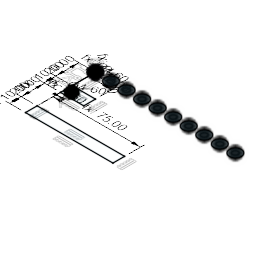
Initial_Gears (Autodesk Fusion 360 design; units mm, degrees)
part number: 2026-02-16-14-12-18-314
Autodesk Fusion 360 part; units mm, degrees
(part 1 of 40)
sketch "Crank Slider 2" plane through (0, 0, 0) normal (0, 1, 0) x (1, 0, 0)
  circle A0 centre (0, 0) radius 60
  circle A1 centre (0, 0) radius 50 construction
  line L0 (0, 0) -> (0, 50) construction
  circle A2 centre (0, 50) radius 2.3
  circle A3 centre (0, 0) radius 2.3
  line L1 (0, 0) -> (100, 0) construction
  line L2 (130, 5) -> (70, 5)
  line L3 (70, 5) -> (70, -5)
  line L4 (70, -5) -> (130, -5)
  line L5 (130, -5) -> (130, 5)
  line L6 (130, 5) -> (70, -5) construction
  line L7 (70, 5) -> (130, -5) construction
  line L8 (100, 0) -> (75, 0) construction
  line L9 (100, 0) -> (125, 0) construction
  circle A4 centre (75, 0) radius 2.3
  circle A5 centre (125, 0) radius 2.3
  line L10 (100, 0) -> (250, 0) construction
  line L11 (330, 5) -> (170, 5)
  line L12 (170, 5) -> (170, -5)
  line L13 (170, -5) -> (330, -5)
  line L14 (330, -5) -> (330, 5)
  line L15 (330, 5) -> (170, -5) construction
  line L16 (170, 5) -> (330, -5) construction
  line L17 (250, 0) -> (175, 0) construction
  line L18 (250, 0) -> (325, 0) construction
  circle A6 centre (175, 0) radius 2.3
  circle A7 centre (325, 0) radius 2.3
  line L19 (325, 0) -> (375, 0) construction
  line L20 (365, 5) -> (385, 5)
  line L21 (385, 5) -> (385, -5)
  line L22 (385, -5) -> (365, -5)
  line L23 (365, -5) -> (365, 5)
  line L24 (365, 5) -> (385, -5) construction
  line L25 (385, 5) -> (365, -5) construction
  line L26 (375, 0) -> (525, 0) construction
  line L27 (637.5, 5) -> (412.5, 5)
  line L28 (412.5, 5) -> (412.5, -5)
  line L29 (412.5, -5) -> (637.5, -5)
  line L30 (637.5, -5) -> (637.5, 5)
  line L31 (637.5, 5) -> (412.5, -5) construction
  line L32 (412.5, 5) -> (637.5, -5) construction
  line L33 (412.5, 5) -> (637.5, 5)
  line L34 (637.5, 5) -> (637.5, 15)
  line L35 (637.5, 15) -> (412.5, 15)
  line L36 (412.5, 15) -> (412.5, 5)
  line L37 (412.5, -15) -> (412.5, -5)
  line L38 (637.5, -15) -> (412.5, -15)
  line L39 (637.5, -5) -> (637.5, -15)
  circle A8 centre (375, 0) radius 2.3
  line L40 (271.0638, 125.2182) -> (271.2213, 125.2035) construction
  line L41 (271.2213, 125.2035) -> (271.3791, 125.1902) construction
  point P0 (100, 0)
  point P1 (250, 0)
  point P2 (375, 0)
  point P3 (525, 0)
  dimension "d1" = 120
  dimension "d4" = 100
  dimension "d6" = 4.6
  dimension "d7" = 4.6
  dimension "d8" = 100
  dimension "d11" = 60
  dimension "d12" = 10
  dimension "d13" = 25
  dimension "d14" = 25
  dimension "d15" = 4.6
  dimension "d16" = 4.6
  dimension "d18" = 150
  dimension "d20" = 160
  dimension "d21" = 10
  dimension "d22" = 75
  dimension "d23" = 75
  dimension "d24" = 4.6
  dimension "d25" = 4.6
  dimension "d26" = 50
  dimension "d27" = 20
  dimension "d28" = 10
  dimension "d29" = 150
  dimension "d30" = 225
  dimension "d31" = 10
  dimension "d32" = 225
  dimension "d33" = 10
  dimension "d34" = 4.6
  constraint coincident A0.centre A1.centre
  constraint coincident A1 L0.end
  constraint vertical L0
  constraint coincident L0.end A2.centre
  constraint concentric A0 A3
  constraint perpendicular L0 L1
  constraint horizontal L2
  constraint perpendicular L2 L3
  constraint parallel L2 L4
  constraint parallel L3 L5
  constraint coincident L6 P0
  constraint coincident L7 P0
  constraint coincident P0 L1.end
  constraint parallel L1 L8
  constraint parallel L8 L9
  constraint coincident L8.end A4.centre
  constraint coincident L9.end A5.centre
  constraint parallel L9 L10
  constraint horizontal L11
  constraint perpendicular L11 L12
  constraint parallel L11 L13
  constraint parallel L12 L14
  constraint coincident L15 P1
  constraint coincident L16 P1
  constraint coincident P1 L10.end
  constraint parallel L10 L17
  constraint parallel L10 L18
  constraint coincident L17.end A6.centre
  constraint coincident L18.end A7.centre
  constraint parallel L18 L19
  constraint horizontal L20
  constraint perpendicular L20 L21
  constraint parallel L20 L22
  constraint parallel L21 L23
  constraint coincident L24 P2
  constraint coincident L25 P2
  constraint coincident P2 L19.end
  constraint perpendicular L21 L26
  constraint horizontal L27
  constraint perpendicular L27 L28
  constraint parallel L27 L29
  constraint parallel L28 L30
  constraint coincident L31 P3
  constraint coincident L32 P3
  constraint coincident P3 L26.end
  constraint horizontal L33
  constraint vertical L34
  constraint horizontal L35
  constraint vertical L36
  constraint symmetric L26 L27.end L28.end
  constraint symmetric L26 L27.start L29.end
  constraint symmetric L26 L34.end L38.start
  constraint symmetric L26 L35.end L37.start
  measures "d1" diameter of A0
  measures "d4" diameter of A1
  measures "d6" diameter of A2
  measures "d7" diameter of A3
  measures "d8" distance of A0.centre P0
  measures "d11" distance of L3.end L4.end
  measures "d12" distance of L2.end L3.end
  measures "d13" distance of P0 L8.end
  measures "d14" distance of P0 L9.end
  measures "d15" diameter of A4
  measures "d16" diameter of A5
  measures "d18" distance of P0 P1
  measures "d20" distance of L12.end L13.end
  measures "d21" distance of L11.end L12.end
  measures "d22" distance of P1 L17.end
  measures "d23" distance of P1 L18.end
  measures "d24" diameter of A6
  measures "d25" diameter of A7
  measures "d26" distance of L18.end P2
  measures "d27" distance of L21.end L22.end
  measures "d28" distance of L20.end L21.end
  measures "d29" distance of P2 P3
  measures "d30" distance of L28.end L29.end
  measures "d31" distance of L27.end L28.end
  measures "d32" distance of L27.end L27.start
  measures "d33" distance of L27.end L35.end
  measures "d34" diameter of A8
extrude "Extrude1" add sketch "Crank Slider 2" along normal blind 4.2 makes body 1 at (274.7199, 0, 4.047) makes body 2 at (108.0532, 0, -4.047) makes body 3 at (367.5667, 0, 0) makes body 4 at (-13.4258, 0, -32.3033) makes body 5 at (487.5, 0, 5)
sketch "Sketch2" plane through (0, 0, 0) normal (0, 1, 0) x (1, 0, 0)
  line L0 (0, 0) -> (212.132, 0) construction
  line L1 (212.132, 0) -> (212.132, 150) construction
  line L2 (212.132, 150) -> (0, 0) construction
  line L3 (0, 0) -> (-50, 0) construction
  line L4 (-50, 0) -> (-50, -100) construction
  line L5 (-50, -100) -> (250, -100)
  line L6 (250, -100) -> (250, 200)
  line L7 (250, 200) -> (-50, 200)
  line L8 (-50, 200) -> (-50, -100)
  circle A0 centre (212.132, 150) radius 2.3
  circle A1 centre (212.132, 0) radius 2.3
  circle A2 centre (0, 0) radius 2.3
  line L9 (0, 0) -> (106.066, 75) construction
  circle A3 centre (106.066, 75) radius 2.3
  dimension "d41" = 212.132
  dimension "d42" = 150
  dimension "d43" = 259.8076
  dimension "d44" = 50
  dimension "d45" = 100
  dimension "d46" = 300
  dimension "d47" = 300
  dimension "d48" = 4.6
  dimension "d49" = 4.6
  dimension "d50" = 4.6
  dimension "d74" = 4.6
  constraint coincident L0.start L2.end
  constraint horizontal L0
  constraint perpendicular L0 L1
  constraint parallel L0 L3
  constraint perpendicular L3 L4
  constraint horizontal L5
  constraint vertical L6
  constraint horizontal L7
  constraint vertical L8
  constraint coincident L1.end L2.start
  constraint coincident L0.end L1.start
  constraint midpoint L2 L9.end
  constraint coincident L9.end A3.centre
  measures "d41" distance of L0.start L0.end
  measures "d42" distance of L0.end L1.end
  measures "d43" distance of L1.end L0.start
  measures "d44" distance of L0.start L3.end
  measures "d45" distance of L3.end L4.end
  measures "d46" distance of L4.end L5.end
  measures "d47" distance of L4.end L7.end
  measures "d48" diameter of A0
  measures "d49" diameter of A1
  measures "d50" diameter of A2
  measures "d74" diameter of A3
sketch "Sketch3" plane through (0, 0, 0) normal (0, 1, 0) x (1, 0, 0)
  line L0 (212.132, 150) -> (0, 0) construction
  line L1 (0, 0) -> (212.132, 0) construction
  line L2 (212.132, 0) -> (212.132, 150) construction
  line L3 (0, 0) -> (0, -50) construction
  spline S0 degree 5 poles (166.3167, 109.6737) (166.2935, 109.6533) (166.2466, 109.6132) (166.1747, 109.5549) (166.076, 109.4808) (165.9487, 109.3934) (165.8185, 109.3096) (165.6866, 109.228) (165.5538, 109.1476) (165.4203, 109.068) (165.2862, 108.9893) (165.1513, 108.9117) (165.0152, 108.8358) (164.8777, 108.7617) (164.739, 108.6894) (164.5991, 108.6187) (164.4582, 108.5496) (164.3164, 108.4816) (164.1739, 108.4147) (164.0308, 108.3488) (163.887, 108.284) (163.7425, 108.2202) (163.5973, 108.1576) (163.4513, 108.0961) (163.3046, 108.0358) (163.1571, 107.9766) (163.009, 107.9185) (162.8603, 107.8614) (162.711, 107.8053) (162.5611, 107.7501) (162.4106, 107.6959) (162.2596, 107.6426) (162.108, 107.5903) (161.9559, 107.539) (161.8032, 107.4886) (161.65, 107.4392) (161.4962, 107.3906) (161.342, 107.343) (161.1873, 107.2963) (161.0321, 107.2505) (160.8764, 107.2055) (160.7202, 107.1614) (160.5636, 107.1182) (160.4065, 107.0759) (160.249, 107.0344) (160.0911, 106.9937) (159.9327, 106.9539) (159.7739, 106.915) (159.6147, 106.8769) (159.4551, 106.8396) (159.2951, 106.8031) (159.1347, 106.7674) (158.9739, 106.7326) (158.8127, 106.6985) (158.6511, 106.6653) (158.4892, 106.6328) (158.3269, 106.6012) (158.1643, 106.5703) (158.0013, 106.5403) (157.838, 106.511) (157.6743, 106.4825) (157.5103, 106.4547) (157.3459, 106.4277) (157.1812, 106.4016) (157.0162, 106.3761) (156.8509, 106.3514) (156.6853, 106.3275) (156.5194, 106.3044) (156.3531, 106.282) (156.1866, 106.2603) (156.0198, 106.2394) (155.8861, 106.2233) (155.7857, 106.2115) (155.7187, 106.2038) (155.6851, 106.2) knots 0 0 0 0 0 0 0.01428571 0.02857143 0.04285714 0.05714286 0.07142857 0.08571429 0.1 0.11428571 0.12857143 0.14285714 0.15714286 0.17142857 0.18571429 0.2 0.21428571 0.22857143 0.24285714 0.25714286 0.27142857 0.28571429 0.3 0.31428571 0.32857143 0.34285714 0.35714286 0.37142857 0.38571429 0.4 0.41428571 0.42857143 0.44285714 0.45714286 0.47142857 0.48571429 0.5 0.51428571 0.52857143 0.54285714 0.55714286 0.57142857 0.58571429 0.6 0.61428571 0.62857143 0.64285714 0.65714286 0.67142857 0.68571429 0.7 0.71428571 0.72857143 0.74285714 0.75714286 0.77142857 0.78571429 0.8 0.81428571 0.82857143 0.84285714 0.85714286 0.87142857 0.88571429 0.9 0.91428571 0.92857143 0.94285714 0.95714286 0.97142857 0.98571429 1 1 1 1 1 1
  line L4 (166.3167, 109.6737) -> (166.2935, 109.6533) construction
  line L5 (166.2935, 109.6533) -> (166.2466, 109.6132) construction
  line L6 (166.2466, 109.6132) -> (166.1747, 109.5549) construction
  line L7 (166.1747, 109.5549) -> (166.076, 109.4808) construction
  line L8 (166.076, 109.4808) -> (165.9487, 109.3934) construction
  line L9 (165.9487, 109.3934) -> (165.8185, 109.3096) construction
  line L10 (165.8185, 109.3096) -> (165.6866, 109.228) construction
  line L11 (165.6866, 109.228) -> (165.5538, 109.1476) construction
  line L12 (165.5538, 109.1476) -> (165.4203, 109.068) construction
  line L13 (165.4203, 109.068) -> (165.2862, 108.9893) construction
  line L14 (165.2862, 108.9893) -> (165.1513, 108.9117) construction
  line L15 (165.1513, 108.9117) -> (165.0152, 108.8358) construction
  line L16 (165.0152, 108.8358) -> (164.8777, 108.7617) construction
  line L17 (164.8777, 108.7617) -> (164.739, 108.6894) construction
  line L18 (164.739, 108.6894) -> (164.5991, 108.6187) construction
  line L19 (164.5991, 108.6187) -> (164.4582, 108.5496) construction
  line L20 (164.4582, 108.5496) -> (164.3164, 108.4816) construction
  line L21 (164.3164, 108.4816) -> (164.1739, 108.4147) construction
  line L22 (164.1739, 108.4147) -> (164.0308, 108.3488) construction
  line L23 (164.0308, 108.3488) -> (163.887, 108.284) construction
  line L24 (163.887, 108.284) -> (163.7425, 108.2202) construction
  line L25 (163.7425, 108.2202) -> (163.5973, 108.1576) construction
  line L26 (163.5973, 108.1576) -> (163.4513, 108.0961) construction
  line L27 (163.4513, 108.0961) -> (163.3046, 108.0358) construction
  line L28 (163.3046, 108.0358) -> (163.1571, 107.9766) construction
  line L29 (163.1571, 107.9766) -> (163.009, 107.9185) construction
  line L30 (163.009, 107.9185) -> (162.8603, 107.8614) construction
  line L31 (162.8603, 107.8614) -> (162.711, 107.8053) construction
  line L32 (162.711, 107.8053) -> (162.5611, 107.7501) construction
  line L33 (162.5611, 107.7501) -> (162.4106, 107.6959) construction
  line L34 (162.4106, 107.6959) -> (162.2596, 107.6426) construction
  line L35 (162.2596, 107.6426) -> (162.108, 107.5903) construction
  line L36 (162.108, 107.5903) -> (161.9559, 107.539) construction
  line L37 (161.9559, 107.539) -> (161.8032, 107.4886) construction
  line L38 (161.8032, 107.4886) -> (161.65, 107.4392) construction
  line L39 (161.65, 107.4392) -> (161.4962, 107.3906) construction
  line L40 (161.4962, 107.3906) -> (161.342, 107.343) construction
  line L41 (161.342, 107.343) -> (161.1873, 107.2963) construction
  line L42 (161.1873, 107.2963) -> (161.0321, 107.2505) construction
  line L43 (161.0321, 107.2505) -> (160.8764, 107.2055) construction
  line L44 (160.8764, 107.2055) -> (160.7202, 107.1614) construction
  line L45 (160.7202, 107.1614) -> (160.5636, 107.1182) construction
  line L46 (160.5636, 107.1182) -> (160.4065, 107.0759) construction
  line L47 (160.4065, 107.0759) -> (160.249, 107.0344) construction
  line L48 (160.249, 107.0344) -> (160.0911, 106.9937) construction
  line L49 (160.0911, 106.9937) -> (159.9327, 106.9539) construction
  line L50 (159.9327, 106.9539) -> (159.7739, 106.915) construction
  line L51 (159.7739, 106.915) -> (159.6147, 106.8769) construction
  line L52 (159.6147, 106.8769) -> (159.4551, 106.8396) construction
  line L53 (159.4551, 106.8396) -> (159.2951, 106.8031) construction
  line L54 (159.2951, 106.8031) -> (159.1347, 106.7674) construction
  line L55 (159.1347, 106.7674) -> (158.9739, 106.7326) construction
  line L56 (158.9739, 106.7326) -> (158.8127, 106.6985) construction
  line L57 (158.8127, 106.6985) -> (158.6511, 106.6653) construction
  line L58 (158.6511, 106.6653) -> (158.4892, 106.6328) construction
  line L59 (158.4892, 106.6328) -> (158.3269, 106.6012) construction
  line L60 (158.3269, 106.6012) -> (158.1643, 106.5703) construction
  line L61 (158.1643, 106.5703) -> (158.0013, 106.5403) construction
  line L62 (158.0013, 106.5403) -> (157.838, 106.511) construction
  line L63 (157.838, 106.511) -> (157.6743, 106.4825) construction
  line L64 (157.6743, 106.4825) -> (157.5103, 106.4547) construction
  line L65 (157.5103, 106.4547) -> (157.3459, 106.4277) construction
  line L66 (157.3459, 106.4277) -> (157.1812, 106.4016) construction
  line L67 (157.1812, 106.4016) -> (157.0162, 106.3761) construction
  line L68 (157.0162, 106.3761) -> (156.8509, 106.3514) construction
  line L69 (156.8509, 106.3514) -> (156.6853, 106.3275) construction
  line L70 (156.6853, 106.3275) -> (156.5194, 106.3044) construction
  line L71 (156.5194, 106.3044) -> (156.3531, 106.282) construction
  line L72 (156.3531, 106.282) -> (156.1866, 106.2603) construction
  line L73 (156.1866, 106.2603) -> (156.0198, 106.2394) construction
  line L74 (156.0198, 106.2394) -> (155.8861, 106.2233) construction
  line L75 (155.8861, 106.2233) -> (155.7857, 106.2115) construction
  line L76 (155.7857, 106.2115) -> (155.7187, 106.2038) construction
  line L77 (155.7187, 106.2038) -> (155.6851, 106.2) construction
  arc A0 (255.932, 206.4469) -> (252.2812, 209.0993) centre (212.132, 150) ccw
  spline S1 degree 5 poles (166.3167, 190.3263) (166.2935, 190.3467) (166.2466, 190.3868) (166.1747, 190.4451) (166.076, 190.5192) (165.9487, 190.6066) (165.8185, 190.6904) (165.6866, 190.772) (165.5538, 190.8524) (165.4203, 190.932) (165.2862, 191.0107) (165.1513, 191.0883) (165.0152, 191.1642) (164.8777, 191.2383) (164.739, 191.3106) (164.5991, 191.3813) (164.4582, 191.4504) (164.3164, 191.5184) (164.1739, 191.5853) (164.0308, 191.6512) (163.887, 191.716) (163.7425, 191.7798) (163.5973, 191.8424) (163.4513, 191.9039) (163.3046, 191.9642) (163.1571, 192.0234) (163.009, 192.0815) (162.8603, 192.1386) (162.711, 192.1947) (162.5611, 192.2499) (162.4106, 192.3041) (162.2596, 192.3574) (162.108, 192.4097) (161.9559, 192.461) (161.8032, 192.5114) (161.65, 192.5608) (161.4962, 192.6094) (161.342, 192.657) (161.1873, 192.7037) (161.0321, 192.7495) (160.8764, 192.7945) (160.7202, 192.8386) (160.5636, 192.8818) (160.4065, 192.9241) (160.249, 192.9656) (160.0911, 193.0063) (159.9327, 193.0461) (159.7739, 193.085) (159.6147, 193.1231) (159.4551, 193.1604) (159.2951, 193.1969) (159.1347, 193.2326) (158.9739, 193.2674) (158.8127, 193.3015) (158.6511, 193.3347) (158.4892, 193.3672) (158.3269, 193.3988) (158.1643, 193.4297) (158.0013, 193.4597) (157.838, 193.489) (157.6743, 193.5175) (157.5103, 193.5453) (157.3459, 193.5723) (157.1812, 193.5984) (157.0162, 193.6239) (156.8509, 193.6486) (156.6853, 193.6725) (156.5194, 193.6956) (156.3531, 193.718) (156.1866, 193.7397) (156.0198, 193.7606) (155.8861, 193.7767) (155.7857, 193.7885) (155.7187, 193.7962) (155.6851, 193.8) knots 0 0 0 0 0 0 0.01428571 0.02857143 0.04285714 0.05714286 0.07142857 0.08571429 0.1 0.11428571 0.12857143 0.14285714 0.15714286 0.17142857 0.18571429 0.2 0.21428571 0.22857143 0.24285714 0.25714286 0.27142857 0.28571429 0.3 0.31428571 0.32857143 0.34285714 0.35714286 0.37142857 0.38571429 0.4 0.41428571 0.42857143 0.44285714 0.45714286 0.47142857 0.48571429 0.5 0.51428571 0.52857143 0.54285714 0.55714286 0.57142857 0.58571429 0.6 0.61428571 0.62857143 0.64285714 0.65714286 0.67142857 0.68571429 0.7 0.71428571 0.72857143 0.74285714 0.75714286 0.77142857 0.78571429 0.8 0.81428571 0.82857143 0.84285714 0.85714286 0.87142857 0.88571429 0.9 0.91428571 0.92857143 0.94285714 0.95714286 0.97142857 0.98571429 1 1 1 1 1 1
  line L78 (166.3167, 190.3263) -> (166.2935, 190.3467) construction
  line L79 (166.2935, 190.3467) -> (166.2466, 190.3868) construction
  line L80 (166.2466, 190.3868) -> (166.1747, 190.4451) construction
  line L81 (166.1747, 190.4451) -> (166.076, 190.5192) construction
  line L82 (166.076, 190.5192) -> (165.9487, 190.6066) construction
  line L83 (165.9487, 190.6066) -> (165.8185, 190.6904) construction
  line L84 (165.8185, 190.6904) -> (165.6866, 190.772) construction
  line L85 (165.6866, 190.772) -> (165.5538, 190.8524) construction
  line L86 (165.5538, 190.8524) -> (165.4203, 190.932) construction
  line L87 (165.4203, 190.932) -> (165.2862, 191.0107) construction
  line L88 (165.2862, 191.0107) -> (165.1513, 191.0883) construction
  line L89 (165.1513, 191.0883) -> (165.0152, 191.1642) construction
  line L90 (165.0152, 191.1642) -> (164.8777, 191.2383) construction
  line L91 (164.8777, 191.2383) -> (164.739, 191.3106) construction
  line L92 (164.739, 191.3106) -> (164.5991, 191.3813) construction
  line L93 (164.5991, 191.3813) -> (164.4582, 191.4504) construction
  line L94 (164.4582, 191.4504) -> (164.3164, 191.5184) construction
  line L95 (164.3164, 191.5184) -> (164.1739, 191.5853) construction
  line L96 (164.1739, 191.5853) -> (164.0308, 191.6512) construction
  line L97 (164.0308, 191.6512) -> (163.887, 191.716) construction
  line L98 (163.887, 191.716) -> (163.7425, 191.7798) construction
  line L99 (163.7425, 191.7798) -> (163.5973, 191.8424) construction
  line L100 (163.5973, 191.8424) -> (163.4513, 191.9039) construction
  line L101 (163.4513, 191.9039) -> (163.3046, 191.9642) construction
  line L102 (163.3046, 191.9642) -> (163.1571, 192.0234) construction
  line L103 (163.1571, 192.0234) -> (163.009, 192.0815) construction
  line L104 (163.009, 192.0815) -> (162.8603, 192.1386) construction
  line L105 (162.8603, 192.1386) -> (162.711, 192.1947) construction
  line L106 (162.711, 192.1947) -> (162.5611, 192.2499) construction
  line L107 (162.5611, 192.2499) -> (162.4106, 192.3041) construction
  line L108 (162.4106, 192.3041) -> (162.2596, 192.3574) construction
  line L109 (162.2596, 192.3574) -> (162.108, 192.4097) construction
  line L110 (162.108, 192.4097) -> (161.9559, 192.461) construction
  line L111 (161.9559, 192.461) -> (161.8032, 192.5114) construction
  line L112 (161.8032, 192.5114) -> (161.65, 192.5608) construction
  line L113 (161.65, 192.5608) -> (161.4962, 192.6094) construction
  line L114 (161.4962, 192.6094) -> (161.342, 192.657) construction
  line L115 (161.342, 192.657) -> (161.1873, 192.7037) construction
  line L116 (161.1873, 192.7037) -> (161.0321, 192.7495) construction
  line L117 (161.0321, 192.7495) -> (160.8764, 192.7945) construction
  line L118 (160.8764, 192.7945) -> (160.7202, 192.8386) construction
  line L119 (160.7202, 192.8386) -> (160.5636, 192.8818) construction
  line L120 (160.5636, 192.8818) -> (160.4065, 192.9241) construction
  line L121 (160.4065, 192.9241) -> (160.249, 192.9656) construction
  line L122 (160.249, 192.9656) -> (160.0911, 193.0063) construction
  line L123 (160.0911, 193.0063) -> (159.9327, 193.0461) construction
  line L124 (159.9327, 193.0461) -> (159.7739, 193.085) construction
  line L125 (159.7739, 193.085) -> (159.6147, 193.1231) construction
  line L126 (159.6147, 193.1231) -> (159.4551, 193.1604) construction
  line L127 (159.4551, 193.1604) -> (159.2951, 193.1969) construction
  line L128 (159.2951, 193.1969) -> (159.1347, 193.2326) construction
  line L129 (159.1347, 193.2326) -> (158.9739, 193.2674) construction
  line L130 (158.9739, 193.2674) -> (158.8127, 193.3015) construction
  line L131 (158.8127, 193.3015) -> (158.6511, 193.3347) construction
  line L132 (158.6511, 193.3347) -> (158.4892, 193.3672) construction
  line L133 (158.4892, 193.3672) -> (158.3269, 193.3988) construction
  line L134 (158.3269, 193.3988) -> (158.1643, 193.4297) construction
  line L135 (158.1643, 193.4297) -> (158.0013, 193.4597) construction
  line L136 (158.0013, 193.4597) -> (157.838, 193.489) construction
  line L137 (157.838, 193.489) -> (157.6743, 193.5175) construction
  line L138 (157.6743, 193.5175) -> (157.5103, 193.5453) construction
  line L139 (157.5103, 193.5453) -> (157.3459, 193.5723) construction
  line L140 (157.3459, 193.5723) -> (157.1812, 193.5984) construction
  line L141 (157.1812, 193.5984) -> (157.0162, 193.6239) construction
  line L142 (157.0162, 193.6239) -> (156.8509, 193.6486) construction
  line L143 (156.8509, 193.6486) -> (156.6853, 193.6725) construction
  line L144 (156.6853, 193.6725) -> (156.5194, 193.6956) construction
  line L145 (156.5194, 193.6956) -> (156.3531, 193.718) construction
  line L146 (156.3531, 193.718) -> (156.1866, 193.7397) construction
  line L147 (156.1866, 193.7397) -> (156.0198, 193.7606) construction
  line L148 (156.0198, 193.7606) -> (155.8861, 193.7767) construction
  line L149 (155.8861, 193.7767) -> (155.7857, 193.7885) construction
  line L150 (155.7857, 193.7885) -> (155.7187, 193.7962) construction
  line L151 (155.7187, 193.7962) -> (155.6851, 193.8) construction
  spline S2 degree 5 poles (166.3167, 109.6737) (166.2935, 109.6533) (166.2466, 109.6132) (166.1747, 109.5549) (166.076, 109.4808) (165.9487, 109.3934) (165.8185, 109.3096) (165.6866, 109.228) (165.5538, 109.1476) (165.4203, 109.068) (165.2862, 108.9893) (165.1513, 108.9117) (165.0152, 108.8358) (164.8777, 108.7617) (164.739, 108.6894) (164.5991, 108.6187) (164.4582, 108.5496) (164.3164, 108.4816) (164.1739, 108.4147) (164.0308, 108.3488) (163.887, 108.284) (163.7425, 108.2202) (163.5973, 108.1576) (163.4513, 108.0961) (163.3046, 108.0358) (163.1571, 107.9766) (163.009, 107.9185) (162.8603, 107.8614) (162.711, 107.8053) (162.5611, 107.7501) (162.4106, 107.6959) (162.2596, 107.6426) (162.108, 107.5903) (161.9559, 107.539) (161.8032, 107.4886) (161.65, 107.4392) (161.4962, 107.3906) (161.342, 107.343) (161.1873, 107.2963) (161.0321, 107.2505) (160.8764, 107.2055) (160.7202, 107.1614) (160.5636, 107.1182) (160.4065, 107.0759) (160.249, 107.0344) (160.0911, 106.9937) (159.9327, 106.9539) (159.7739, 106.915) (159.6147, 106.8769) (159.4551, 106.8396) (159.2951, 106.8031) (159.1347, 106.7674) (158.9739, 106.7326) (158.8127, 106.6985) (158.6511, 106.6653) (158.4892, 106.6328) (158.3269, 106.6012) (158.1643, 106.5703) (158.0013, 106.5403) (157.838, 106.511) (157.6743, 106.4825) (157.5103, 106.4547) (157.3459, 106.4277) (157.1812, 106.4016) (157.0162, 106.3761) (156.8509, 106.3514) (156.6853, 106.3275) (156.5194, 106.3044) (156.3531, 106.282) (156.1866, 106.2603) (156.0198, 106.2394) (155.8861, 106.2233) (155.7857, 106.2115) (155.7187, 106.2038) (155.6851, 106.2) knots 0 0 0 0 0 0 0.01428571 0.02857143 0.04285714 0.05714286 0.07142857 0.08571429 0.1 0.11428571 0.12857143 0.14285714 0.15714286 0.17142857 0.18571429 0.2 0.21428571 0.22857143 0.24285714 0.25714286 0.27142857 0.28571429 0.3 0.31428571 0.32857143 0.34285714 0.35714286 0.37142857 0.38571429 0.4 0.41428571 0.42857143 0.44285714 0.45714286 0.47142857 0.48571429 0.5 0.51428571 0.52857143 0.54285714 0.55714286 0.57142857 0.58571429 0.6 0.61428571 0.62857143 0.64285714 0.65714286 0.67142857 0.68571429 0.7 0.71428571 0.72857143 0.74285714 0.75714286 0.77142857 0.78571429 0.8 0.81428571 0.82857143 0.84285714 0.85714286 0.87142857 0.88571429 0.9 0.91428571 0.92857143 0.94285714 0.95714286 0.97142857 0.98571429 1 1 1 1 1 1
  line L152 (166.3167, 109.6737) -> (166.2935, 109.6533) construction
  line L153 (166.2935, 109.6533) -> (166.2466, 109.6132) construction
  line L154 (166.2466, 109.6132) -> (166.1747, 109.5549) construction
  line L155 (166.1747, 109.5549) -> (166.076, 109.4808) construction
  line L156 (166.076, 109.4808) -> (165.9487, 109.3934) construction
  line L157 (165.9487, 109.3934) -> (165.8185, 109.3096) construction
  line L158 (165.8185, 109.3096) -> (165.6866, 109.228) construction
  line L159 (165.6866, 109.228) -> (165.5538, 109.1476) construction
  line L160 (165.5538, 109.1476) -> (165.4203, 109.068) construction
  line L161 (165.4203, 109.068) -> (165.2862, 108.9893) construction
  line L162 (165.2862, 108.9893) -> (165.1513, 108.9117) construction
  line L163 (165.1513, 108.9117) -> (165.0152, 108.8358) construction
  line L164 (165.0152, 108.8358) -> (164.8777, 108.7617) construction
  line L165 (164.8777, 108.7617) -> (164.739, 108.6894) construction
  line L166 (164.739, 108.6894) -> (164.5991, 108.6187) construction
  line L167 (164.5991, 108.6187) -> (164.4582, 108.5496) construction
  line L168 (164.4582, 108.5496) -> (164.3164, 108.4816) construction
  line L169 (164.3164, 108.4816) -> (164.1739, 108.4147) construction
  line L170 (164.1739, 108.4147) -> (164.0308, 108.3488) construction
  line L171 (164.0308, 108.3488) -> (163.887, 108.284) construction
  line L172 (163.887, 108.284) -> (163.7425, 108.2202) construction
  line L173 (163.7425, 108.2202) -> (163.5973, 108.1576) construction
  line L174 (163.5973, 108.1576) -> (163.4513, 108.0961) construction
  line L175 (163.4513, 108.0961) -> (163.3046, 108.0358) construction
  line L176 (163.3046, 108.0358) -> (163.1571, 107.9766) construction
  line L177 (163.1571, 107.9766) -> (163.009, 107.9185) construction
  line L178 (163.009, 107.9185) -> (162.8603, 107.8614) construction
  line L179 (162.8603, 107.8614) -> (162.711, 107.8053) construction
  line L180 (162.711, 107.8053) -> (162.5611, 107.7501) construction
  line L181 (162.5611, 107.7501) -> (162.4106, 107.6959) construction
  line L182 (162.4106, 107.6959) -> (162.2596, 107.6426) construction
  line L183 (162.2596, 107.6426) -> (162.108, 107.5903) construction
  line L184 (162.108, 107.5903) -> (161.9559, 107.539) construction
  line L185 (161.9559, 107.539) -> (161.8032, 107.4886) construction
  line L186 (161.8032, 107.4886) -> (161.65, 107.4392) construction
  line L187 (161.65, 107.4392) -> (161.4962, 107.3906) construction
  line L188 (161.4962, 107.3906) -> (161.342, 107.343) construction
  line L189 (161.342, 107.343) -> (161.1873, 107.2963) construction
  line L190 (161.1873, 107.2963) -> (161.0321, 107.2505) construction
  line L191 (161.0321, 107.2505) -> (160.8764, 107.2055) construction
  line L192 (160.8764, 107.2055) -> (160.7202, 107.1614) construction
  line L193 (160.7202, 107.1614) -> (160.5636, 107.1182) construction
  line L194 (160.5636, 107.1182) -> (160.4065, 107.0759) construction
  line L195 (160.4065, 107.0759) -> (160.249, 107.0344) construction
  line L196 (160.249, 107.0344) -> (160.0911, 106.9937) construction
  line L197 (160.0911, 106.9937) -> (159.9327, 106.9539) construction
  line L198 (159.9327, 106.9539) -> (159.7739, 106.915) construction
  line L199 (159.7739, 106.915) -> (159.6147, 106.8769) construction
  line L200 (159.6147, 106.8769) -> (159.4551, 106.8396) construction
  line L201 (159.4551, 106.8396) -> (159.2951, 106.8031) construction
  line L202 (159.2951, 106.8031) -> (159.1347, 106.7674) construction
  line L203 (159.1347, 106.7674) -> (158.9739, 106.7326) construction
  line L204 (158.9739, 106.7326) -> (158.8127, 106.6985) construction
  line L205 (158.8127, 106.6985) -> (158.6511, 106.6653) construction
  line L206 (158.6511, 106.6653) -> (158.4892, 106.6328) construction
  line L207 (158.4892, 106.6328) -> (158.3269, 106.6012) construction
  line L208 (158.3269, 106.6012) -> (158.1643, 106.5703) construction
  line L209 (158.1643, 106.5703) -> (158.0013, 106.5403) construction
  line L210 (158.0013, 106.5403) -> (157.838, 106.511) construction
  line L211 (157.838, 106.511) -> (157.6743, 106.4825) construction
  line L212 (157.6743, 106.4825) -> (157.5103, 106.4547) construction
  line L213 (157.5103, 106.4547) -> (157.3459, 106.4277) construction
  line L214 (157.3459, 106.4277) -> (157.1812, 106.4016) construction
  line L215 (157.1812, 106.4016) -> (157.0162, 106.3761) construction
  line L216 (157.0162, 106.3761) -> (156.8509, 106.3514) construction
  line L217 (156.8509, 106.3514) -> (156.6853, 106.3275) construction
  line L218 (156.6853, 106.3275) -> (156.5194, 106.3044) construction
  line L219 (156.5194, 106.3044) -> (156.3531, 106.282) construction
  line L220 (156.3531, 106.282) -> (156.1866, 106.2603) construction
  line L221 (156.1866, 106.2603) -> (156.0198, 106.2394) construction
  line L222 (156.0198, 106.2394) -> (155.8861, 106.2233) construction
  line L223 (155.8861, 106.2233) -> (155.7857, 106.2115) construction
  line L224 (155.7857, 106.2115) -> (155.7187, 106.2038) construction
  line L225 (155.7187, 106.2038) -> (155.6851, 106.2) construction
  spline S3 degree 5 poles (166.3167, 190.3263) (166.2935, 190.3467) (166.2466, 190.3868) (166.1747, 190.4451) (166.076, 190.5192) (165.9487, 190.6066) (165.8185, 190.6904) (165.6866, 190.772) (165.5538, 190.8524) (165.4203, 190.932) (165.2862, 191.0107) (165.1513, 191.0883) (165.0152, 191.1642) (164.8777, 191.2383) (164.739, 191.3106) (164.5991, 191.3813) (164.4582, 191.4504) (164.3164, 191.5184) (164.1739, 191.5853) (164.0308, 191.6512) (163.887, 191.716) (163.7425, 191.7798) (163.5973, 191.8424) (163.4513, 191.9039) (163.3046, 191.9642) (163.1571, 192.0234) (163.009, 192.0815) (162.8603, 192.1386) (162.711, 192.1947) (162.5611, 192.2499) (162.4106, 192.3041) (162.2596, 192.3574) (162.108, 192.4097) (161.9559, 192.461) (161.8032, 192.5114) (161.65, 192.5608) (161.4962, 192.6094) (161.342, 192.657) (161.1873, 192.7037) (161.0321, 192.7495) (160.8764, 192.7945) (160.7202, 192.8386) (160.5636, 192.8818) (160.4065, 192.9241) (160.249, 192.9656) (160.0911, 193.0063) (159.9327, 193.0461) (159.7739, 193.085) (159.6147, 193.1231) (159.4551, 193.1604) (159.2951, 193.1969) (159.1347, 193.2326) (158.9739, 193.2674) (158.8127, 193.3015) (158.6511, 193.3347) (158.4892, 193.3672) (158.3269, 193.3988) (158.1643, 193.4297) (158.0013, 193.4597) (157.838, 193.489) (157.6743, 193.5175) (157.5103, 193.5453) (157.3459, 193.5723) (157.1812, 193.5984) (157.0162, 193.6239) (156.8509, 193.6486) (156.6853, 193.6725) (156.5194, 193.6956) (156.3531, 193.718) (156.1866, 193.7397) (156.0198, 193.7606) (155.8861, 193.7767) (155.7857, 193.7885) (155.7187, 193.7962) (155.6851, 193.8) knots 0 0 0 0 0 0 0.01428571 0.02857143 0.04285714 0.05714286 0.07142857 0.08571429 0.1 0.11428571 0.12857143 0.14285714 0.15714286 0.17142857 0.18571429 0.2 0.21428571 0.22857143 0.24285714 0.25714286 0.27142857 0.28571429 0.3 0.31428571 0.32857143 0.34285714 0.35714286 0.37142857 0.38571429 0.4 0.41428571 0.42857143 0.44285714 0.45714286 0.47142857 0.48571429 0.5 0.51428571 0.52857143 0.54285714 0.55714286 0.57142857 0.58571429 0.6 0.61428571 0.62857143 0.64285714 0.65714286 0.67142857 0.68571429 0.7 0.71428571 0.72857143 0.74285714 0.75714286 0.77142857 0.78571429 0.8 0.81428571 0.82857143 0.84285714 0.85714286 0.87142857 0.88571429 0.9 0.91428571 0.92857143 0.94285714 0.95714286 0.97142857 0.98571429 1 1 1 1 1 1
  line L226 (166.3167, 190.3263) -> (166.2935, 190.3467) construction
  line L227 (166.2935, 190.3467) -> (166.2466, 190.3868) construction
  line L228 (166.2466, 190.3868) -> (166.1747, 190.4451) construction
  line L229 (166.1747, 190.4451) -> (166.076, 190.5192) construction
  line L230 (166.076, 190.5192) -> (165.9487, 190.6066) construction
  line L231 (165.9487, 190.6066) -> (165.8185, 190.6904) construction
  line L232 (165.8185, 190.6904) -> (165.6866, 190.772) construction
  line L233 (165.6866, 190.772) -> (165.5538, 190.8524) construction
  line L234 (165.5538, 190.8524) -> (165.4203, 190.932) construction
  line L235 (165.4203, 190.932) -> (165.2862, 191.0107) construction
  line L236 (165.2862, 191.0107) -> (165.1513, 191.0883) construction
  line L237 (165.1513, 191.0883) -> (165.0152, 191.1642) construction
  line L238 (165.0152, 191.1642) -> (164.8777, 191.2383) construction
  line L239 (164.8777, 191.2383) -> (164.739, 191.3106) construction
  line L240 (164.739, 191.3106) -> (164.5991, 191.3813) construction
  line L241 (164.5991, 191.3813) -> (164.4582, 191.4504) construction
  line L242 (164.4582, 191.4504) -> (164.3164, 191.5184) construction
  line L243 (164.3164, 191.5184) -> (164.1739, 191.5853) construction
  line L244 (164.1739, 191.5853) -> (164.0308, 191.6512) construction
  line L245 (164.0308, 191.6512) -> (163.887, 191.716) construction
  line L246 (163.887, 191.716) -> (163.7425, 191.7798) construction
  line L247 (163.7425, 191.7798) -> (163.5973, 191.8424) construction
  line L248 (163.5973, 191.8424) -> (163.4513, 191.9039) construction
  line L249 (163.4513, 191.9039) -> (163.3046, 191.9642) construction
  line L250 (163.3046, 191.9642) -> (163.1571, 192.0234) construction
  line L251 (163.1571, 192.0234) -> (163.009, 192.0815) construction
  line L252 (163.009, 192.0815) -> (162.8603, 192.1386) construction
  line L253 (162.8603, 192.1386) -> (162.711, 192.1947) construction
  line L254 (162.711, 192.1947) -> (162.5611, 192.2499) construction
  line L255 (162.5611, 192.2499) -> (162.4106, 192.3041) construction
  line L256 (162.4106, 192.3041) -> (162.2596, 192.3574) construction
  line L257 (162.2596, 192.3574) -> (162.108, 192.4097) construction
  line L258 (162.108, 192.4097) -> (161.9559, 192.461) construction
  line L259 (161.9559, 192.461) -> (161.8032, 192.5114) construction
  line L260 (161.8032, 192.5114) -> (161.65, 192.5608) construction
  line L261 (161.65, 192.5608) -> (161.4962, 192.6094) construction
  line L262 (161.4962, 192.6094) -> (161.342, 192.657) construction
  line L263 (161.342, 192.657) -> (161.1873, 192.7037) construction
  line L264 (161.1873, 192.7037) -> (161.0321, 192.7495) construction
  line L265 (161.0321, 192.7495) -> (160.8764, 192.7945) construction
  line L266 (160.8764, 192.7945) -> (160.7202, 192.8386) construction
  line L267 (160.7202, 192.8386) -> (160.5636, 192.8818) construction
  line L268 (160.5636, 192.8818) -> (160.4065, 192.9241) construction
  line L269 (160.4065, 192.9241) -> (160.249, 192.9656) construction
  line L270 (160.249, 192.9656) -> (160.0911, 193.0063) construction
  line L271 (160.0911, 193.0063) -> (159.9327, 193.0461) construction
  line L272 (159.9327, 193.0461) -> (159.7739, 193.085) construction
  line L273 (159.7739, 193.085) -> (159.6147, 193.1231) construction
  line L274 (159.6147, 193.1231) -> (159.4551, 193.1604) construction
  line L275 (159.4551, 193.1604) -> (159.2951, 193.1969) construction
  line L276 (159.2951, 193.1969) -> (159.1347, 193.2326) construction
  line L277 (159.1347, 193.2326) -> (158.9739, 193.2674) construction
  line L278 (158.9739, 193.2674) -> (158.8127, 193.3015) construction
  line L279 (158.8127, 193.3015) -> (158.6511, 193.3347) construction
  line L280 (158.6511, 193.3347) -> (158.4892, 193.3672) construction
  line L281 (158.4892, 193.3672) -> (158.3269, 193.3988) construction
  line L282 (158.3269, 193.3988) -> (158.1643, 193.4297) construction
  line L283 (158.1643, 193.4297) -> (158.0013, 193.4597) construction
  line L284 (158.0013, 193.4597) -> (157.838, 193.489) construction
  line L285 (157.838, 193.489) -> (157.6743, 193.5175) construction
  line L286 (157.6743, 193.5175) -> (157.5103, 193.5453) construction
  line L287 (157.5103, 193.5453) -> (157.3459, 193.5723) construction
  line L288 (157.3459, 193.5723) -> (157.1812, 193.5984) construction
  line L289 (157.1812, 193.5984) -> (157.0162, 193.6239) construction
  line L290 (157.0162, 193.6239) -> (156.8509, 193.6486) construction
  line L291 (156.8509, 193.6486) -> (156.6853, 193.6725) construction
  line L292 (156.6853, 193.6725) -> (156.5194, 193.6956) construction
  line L293 (156.5194, 193.6956) -> (156.3531, 193.718) construction
  line L294 (156.3531, 193.718) -> (156.1866, 193.7397) construction
  line L295 (156.1866, 193.7397) -> (156.0198, 193.7606) construction
  line L296 (156.0198, 193.7606) -> (155.8861, 193.7767) construction
  line L297 (155.8861, 193.7767) -> (155.7857, 193.7885) construction
  line L298 (155.7857, 193.7885) -> (155.7187, 193.7962) construction
  line L299 (155.7187, 193.7962) -> (155.6851, 193.8) construction
  arc A1 (253.9452, 189.3784) -> (256.7226, 189.2483) centre (255.4012, 190.7496) ccw
  arc A2 (253.9452, 189.3784) -> (251.5104, 191.8132) centre (212.132, 150) ccw
  line L300 (256.7226, 189.2483) -> (257.9473, 190.3263)
  spline S4 degree 5 poles (257.9473, 190.3263) (257.9705, 190.3467) (258.0174, 190.3868) (258.0893, 190.4451) (258.188, 190.5192) (258.3153, 190.6066) (258.4455, 190.6904) (258.5774, 190.772) (258.7102, 190.8524) (258.8437, 190.932) (258.9778, 191.0107) (259.1127, 191.0883) (259.2488, 191.1642) (259.3863, 191.2383) (259.525, 191.3106) (259.6649, 191.3813) (259.8058, 191.4504) (259.9476, 191.5184) (260.0901, 191.5853) (260.2332, 191.6512) (260.377, 191.716) (260.5215, 191.7798) (260.6667, 191.8424) (260.8127, 191.9039) (260.9594, 191.9642) (261.1069, 192.0234) (261.255, 192.0815) (261.4037, 192.1386) (261.553, 192.1947) (261.7029, 192.2499) (261.8534, 192.3041) (262.0044, 192.3574) (262.156, 192.4097) (262.3081, 192.461) (262.4608, 192.5114) (262.614, 192.5608) (262.7678, 192.6094) (262.922, 192.657) (263.0767, 192.7037) (263.2319, 192.7495) (263.3876, 192.7945) (263.5438, 192.8386) (263.7004, 192.8818) (263.8575, 192.9241) (264.015, 192.9656) (264.1729, 193.0063) (264.3313, 193.0461) (264.4901, 193.085) (264.6493, 193.1231) (264.8089, 193.1604) (264.9689, 193.1969) (265.1293, 193.2326) (265.2901, 193.2674) (265.4513, 193.3015) (265.6129, 193.3347) (265.7748, 193.3672) (265.9371, 193.3988) (266.0997, 193.4297) (266.2627, 193.4597) (266.426, 193.489) (266.5897, 193.5175) (266.7537, 193.5453) (266.9181, 193.5723) (267.0828, 193.5984) (267.2478, 193.6239) (267.4131, 193.6486) (267.5787, 193.6725) (267.7446, 193.6956) (267.9109, 193.718) (268.0774, 193.7397) (268.2442, 193.7606) (268.3779, 193.7767) (268.4783, 193.7885) (268.5453, 193.7962) (268.5789, 193.8) knots 0 0 0 0 0 0 0.01428571 0.02857143 0.04285714 0.05714286 0.07142857 0.08571429 0.1 0.11428571 0.12857143 0.14285714 0.15714286 0.17142857 0.18571429 0.2 0.21428571 0.22857143 0.24285714 0.25714286 0.27142857 0.28571429 0.3 0.31428571 0.32857143 0.34285714 0.35714286 0.37142857 0.38571429 0.4 0.41428571 0.42857143 0.44285714 0.45714286 0.47142857 0.48571429 0.5 0.51428571 0.52857143 0.54285714 0.55714286 0.57142857 0.58571429 0.6 0.61428571 0.62857143 0.64285714 0.65714286 0.67142857 0.68571429 0.7 0.71428571 0.72857143 0.74285714 0.75714286 0.77142857 0.78571429 0.8 0.81428571 0.82857143 0.84285714 0.85714286 0.87142857 0.88571429 0.9 0.91428571 0.92857143 0.94285714 0.95714286 0.97142857 0.98571429 1 1 1 1 1 1
  line L301 (257.9473, 190.3263) -> (257.9705, 190.3467) construction
  line L302 (257.9705, 190.3467) -> (258.0174, 190.3868) construction
  line L303 (258.0174, 190.3868) -> (258.0893, 190.4451) construction
  line L304 (258.0893, 190.4451) -> (258.188, 190.5192) construction
  line L305 (258.188, 190.5192) -> (258.3153, 190.6066) construction
  line L306 (258.3153, 190.6066) -> (258.4455, 190.6904) construction
  line L307 (258.4455, 190.6904) -> (258.5774, 190.772) construction
  line L308 (258.5774, 190.772) -> (258.7102, 190.8524) construction
  line L309 (258.7102, 190.8524) -> (258.8437, 190.932) construction
  line L310 (258.8437, 190.932) -> (258.9778, 191.0107) construction
  line L311 (258.9778, 191.0107) -> (259.1127, 191.0883) construction
  line L312 (259.1127, 191.0883) -> (259.2488, 191.1642) construction
  line L313 (259.2488, 191.1642) -> (259.3863, 191.2383) construction
  line L314 (259.3863, 191.2383) -> (259.525, 191.3106) construction
  line L315 (259.525, 191.3106) -> (259.6649, 191.3813) construction
  line L316 (259.6649, 191.3813) -> (259.8058, 191.4504) construction
  line L317 (259.8058, 191.4504) -> (259.9476, 191.5184) construction
  line L318 (259.9476, 191.5184) -> (260.0901, 191.5853) construction
  line L319 (260.0901, 191.5853) -> (260.2332, 191.6512) construction
  line L320 (260.2332, 191.6512) -> (260.377, 191.716) construction
  line L321 (260.377, 191.716) -> (260.5215, 191.7798) construction
  line L322 (260.5215, 191.7798) -> (260.6667, 191.8424) construction
  line L323 (260.6667, 191.8424) -> (260.8127, 191.9039) construction
  line L324 (260.8127, 191.9039) -> (260.9594, 191.9642) construction
  line L325 (260.9594, 191.9642) -> (261.1069, 192.0234) construction
  line L326 (261.1069, 192.0234) -> (261.255, 192.0815) construction
  line L327 (261.255, 192.0815) -> (261.4037, 192.1386) construction
  line L328 (261.4037, 192.1386) -> (261.553, 192.1947) construction
  line L329 (261.553, 192.1947) -> (261.7029, 192.2499) construction
  line L330 (261.7029, 192.2499) -> (261.8534, 192.3041) construction
  line L331 (261.8534, 192.3041) -> (262.0044, 192.3574) construction
  line L332 (262.0044, 192.3574) -> (262.156, 192.4097) construction
  line L333 (262.156, 192.4097) -> (262.3081, 192.461) construction
  line L334 (262.3081, 192.461) -> (262.4608, 192.5114) construction
  line L335 (262.4608, 192.5114) -> (262.614, 192.5608) construction
  line L336 (262.614, 192.5608) -> (262.7678, 192.6094) construction
  line L337 (262.7678, 192.6094) -> (262.922, 192.657) construction
  line L338 (262.922, 192.657) -> (263.0767, 192.7037) construction
  line L339 (263.0767, 192.7037) -> (263.2319, 192.7495) construction
  line L340 (263.2319, 192.7495) -> (263.3876, 192.7945) construction
  line L341 (263.3876, 192.7945) -> (263.5438, 192.8386) construction
  line L342 (263.5438, 192.8386) -> (263.7004, 192.8818) construction
  line L343 (263.7004, 192.8818) -> (263.8575, 192.9241) construction
  line L344 (263.8575, 192.9241) -> (264.015, 192.9656) construction
  line L345 (264.015, 192.9656) -> (264.1729, 193.0063) construction
  line L346 (264.1729, 193.0063) -> (264.3313, 193.0461) construction
  line L347 (264.3313, 193.0461) -> (264.4901, 193.085) construction
  line L348 (264.4901, 193.085) -> (264.6493, 193.1231) construction
  line L349 (264.6493, 193.1231) -> (264.8089, 193.1604) construction
  line L350 (264.8089, 193.1604) -> (264.9689, 193.1969) construction
  line L351 (264.9689, 193.1969) -> (265.1293, 193.2326) construction
  line L352 (265.1293, 193.2326) -> (265.2901, 193.2674) construction
  line L353 (265.2901, 193.2674) -> (265.4513, 193.3015) construction
  line L354 (265.4513, 193.3015) -> (265.6129, 193.3347) construction
  line L355 (265.6129, 193.3347) -> (265.7748, 193.3672) construction
  line L356 (265.7748, 193.3672) -> (265.9371, 193.3988) construction
  line L357 (265.9371, 193.3988) -> (266.0997, 193.4297) construction
  line L358 (266.0997, 193.4297) -> (266.2627, 193.4597) construction
  line L359 (266.2627, 193.4597) -> (266.426, 193.489) construction
  line L360 (266.426, 193.489) -> (266.5897, 193.5175) construction
  line L361 (266.5897, 193.5175) -> (266.7537, 193.5453) construction
  line L362 (266.7537, 193.5453) -> (266.9181, 193.5723) construction
  line L363 (266.9181, 193.5723) -> (267.0828, 193.5984) construction
  line L364 (267.0828, 193.5984) -> (267.2478, 193.6239) construction
  line L365 (267.2478, 193.6239) -> (267.4131, 193.6486) construction
  line L366 (267.4131, 193.6486) -> (267.5787, 193.6725) construction
  line L367 (267.5787, 193.6725) -> (267.7446, 193.6956) construction
  line L368 (267.7446, 193.6956) -> (267.9109, 193.718) construction
  line L369 (267.9109, 193.718) -> (268.0774, 193.7397) construction
  line L370 (268.0774, 193.7397) -> (268.2442, 193.7606) construction
  line L371 (268.2442, 193.7606) -> (268.3779, 193.7767) construction
  line L372 (268.3779, 193.7767) -> (268.4783, 193.7885) construction
  line L373 (268.4783, 193.7885) -> (268.5453, 193.7962) construction
  line L374 (268.5453, 193.7962) -> (268.5789, 193.8) construction
  spline S5 degree 5 poles (257.9473, 190.3263) (257.9705, 190.3467) (258.0174, 190.3868) (258.0893, 190.4451) (258.188, 190.5192) (258.3153, 190.6066) (258.4455, 190.6904) (258.5774, 190.772) (258.7102, 190.8524) (258.8437, 190.932) (258.9778, 191.0107) (259.1127, 191.0883) (259.2488, 191.1642) (259.3863, 191.2383) (259.525, 191.3106) (259.6649, 191.3813) (259.8058, 191.4504) (259.9476, 191.5184) (260.0901, 191.5853) (260.2332, 191.6512) (260.377, 191.716) (260.5215, 191.7798) (260.6667, 191.8424) (260.8127, 191.9039) (260.9594, 191.9642) (261.1069, 192.0234) (261.255, 192.0815) (261.4037, 192.1386) (261.553, 192.1947) (261.7029, 192.2499) (261.8534, 192.3041) (262.0044, 192.3574) (262.156, 192.4097) (262.3081, 192.461) (262.4608, 192.5114) (262.614, 192.5608) (262.7678, 192.6094) (262.922, 192.657) (263.0767, 192.7037) (263.2319, 192.7495) (263.3876, 192.7945) (263.5438, 192.8386) (263.7004, 192.8818) (263.8575, 192.9241) (264.015, 192.9656) (264.1729, 193.0063) (264.3313, 193.0461) (264.4901, 193.085) (264.6493, 193.1231) (264.8089, 193.1604) (264.9689, 193.1969) (265.1293, 193.2326) (265.2901, 193.2674) (265.4513, 193.3015) (265.6129, 193.3347) (265.7748, 193.3672) (265.9371, 193.3988) (266.0997, 193.4297) (266.2627, 193.4597) (266.426, 193.489) (266.5897, 193.5175) (266.7537, 193.5453) (266.9181, 193.5723) (267.0828, 193.5984) (267.2478, 193.6239) (267.4131, 193.6486) (267.5787, 193.6725) (267.7446, 193.6956) (267.9109, 193.718) (268.0774, 193.7397) (268.2442, 193.7606) (268.3779, 193.7767) (268.4783, 193.7885) (268.5453, 193.7962) (268.5789, 193.8) knots 0 0 0 0 0 0 0.01428571 0.02857143 0.04285714 0.05714286 0.07142857 0.08571429 0.1 0.11428571 0.12857143 0.14285714 0.15714286 0.17142857 0.18571429 0.2 0.21428571 0.22857143 0.24285714 0.25714286 0.27142857 0.28571429 0.3 0.31428571 0.32857143 0.34285714 0.35714286 0.37142857 0.38571429 0.4 0.41428571 0.42857143 0.44285714 0.45714286 0.47142857 0.48571429 0.5 0.51428571 0.52857143 0.54285714 0.55714286 0.57142857 0.58571429 0.6 0.61428571 0.62857143 0.64285714 0.65714286 0.67142857 0.68571429 0.7 0.71428571 0.72857143 0.74285714 0.75714286 0.77142857 0.78571429 0.8 0.81428571 0.82857143 0.84285714 0.85714286 0.87142857 0.88571429 0.9 0.91428571 0.92857143 0.94285714 0.95714286 0.97142857 0.98571429 1 1 1 1 1 1
  line L375 (257.9473, 190.3263) -> (257.9705, 190.3467) construction
  line L376 (257.9705, 190.3467) -> (258.0174, 190.3868) construction
  line L377 (258.0174, 190.3868) -> (258.0893, 190.4451) construction
  line L378 (258.0893, 190.4451) -> (258.188, 190.5192) construction
  line L379 (258.188, 190.5192) -> (258.3153, 190.6066) construction
  line L380 (258.3153, 190.6066) -> (258.4455, 190.6904) construction
  line L381 (258.4455, 190.6904) -> (258.5774, 190.772) construction
  line L382 (258.5774, 190.772) -> (258.7102, 190.8524) construction
  line L383 (258.7102, 190.8524) -> (258.8437, 190.932) construction
  line L384 (258.8437, 190.932) -> (258.9778, 191.0107) construction
  line L385 (258.9778, 191.0107) -> (259.1127, 191.0883) construction
  line L386 (259.1127, 191.0883) -> (259.2488, 191.1642) construction
  line L387 (259.2488, 191.1642) -> (259.3863, 191.2383) construction
  line L388 (259.3863, 191.2383) -> (259.525, 191.3106) construction
  line L389 (259.525, 191.3106) -> (259.6649, 191.3813) construction
  line L390 (259.6649, 191.3813) -> (259.8058, 191.4504) construction
  line L391 (259.8058, 191.4504) -> (259.9476, 191.5184) construction
  line L392 (259.9476, 191.5184) -> (260.0901, 191.5853) construction
  line L393 (260.0901, 191.5853) -> (260.2332, 191.6512) construction
  line L394 (260.2332, 191.6512) -> (260.377, 191.716) construction
  line L395 (260.377, 191.716) -> (260.5215, 191.7798) construction
  line L396 (260.5215, 191.7798) -> (260.6667, 191.8424) construction
  line L397 (260.6667, 191.8424) -> (260.8127, 191.9039) construction
  line L398 (260.8127, 191.9039) -> (260.9594, 191.9642) construction
  line L399 (260.9594, 191.9642) -> (261.1069, 192.0234) construction
  line L400 (261.1069, 192.0234) -> (261.255, 192.0815) construction
  line L401 (261.255, 192.0815) -> (261.4037, 192.1386) construction
  line L402 (261.4037, 192.1386) -> (261.553, 192.1947) construction
  line L403 (261.553, 192.1947) -> (261.7029, 192.2499) construction
  line L404 (261.7029, 192.2499) -> (261.8534, 192.3041) construction